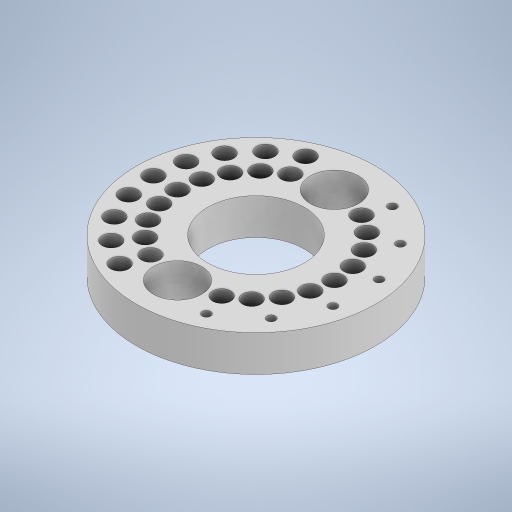
# Autodesk Inventor part: top_housing_wire_guide
Saved by Autodesk Inventor 2023.1 (Build 271208000, 208)
## iProperties
Created: 2026-04-22
Part Number: top_housing_wire_guide
Material: Generic
Document SubType Name: Modeling
Designer: Lars
Density: 1 g/cm^3
Appearance: Default
Author: Lars
Autodesk Inventor part; units mm, degrees
ref_plane "YZ Plane" through (0, 0, 0) normal (1, 0, 0) x (0, 1, 0)
ref_plane "XZ Plane" through (0, 0, 0) normal (0, 1, 0) x (-1, 0, 0)
ref_plane "XY Plane" through (0, 0, 0) normal (0, 0, 1) x (1, 0, 0)
sketch "Sketch2" plane through (0, 0, 0) normal (0, 1, 0) x (-1, 0, 0)
  circle A0 centre (0, 0) radius 10 construction
  circle A1 centre (0, 0) radius 9.9
  circle A2 centre (0, 0) radius 5 construction
  circle A3 centre (0, 0) radius 7 construction
  point P0 (0, 7)
  dimension "d8" = 14
  dimension "d5" = 20
  dimension "d6" = 0.1
  dimension "d7" = 10
  constraints: 3 centre point, 3 coincident, 2 vertical alignment, 2 other
  measures "d5" diameter of A0
  measures "d6" radial gap between concentric circles of A0 A1
  measures "d7" diameter of A2
extrude "Extrusion1" add sketch "Sketch2" along normal blind 3
sketch "Sketch3" plane through (0, 3, 0) normal (0, 1, 0) x (1, 0, 0)
  circle A0 centre (0, 0) radius 6.5 construction
  circle A1 centre (-6.5, 0) radius 0.75
  circle A2 centre (0, 0) radius 4
  circle A3 centre (0, 0) radius 8.5 construction
  circle A4 centre (0, -6.5) radius 2
  circle A5 centre (0, 6.5) radius 2
  circle A6 centre (-6.256, 1.7644) radius 0.75
  circle A7 centre (-5.5422, 3.3962) radius 0.75
  circle A8 centre (-4.4122, 4.7731) radius 0.75
  circle A9 centre (-2.9509, 5.7915) radius 0.75
  circle A10 centre (-6.256, -1.7644) radius 0.75
  circle A11 centre (-5.5422, -3.3962) radius 0.75
  circle A12 centre (-4.4122, -4.7731) radius 0.75
  circle A13 centre (-2.9509, -5.7915) radius 0.75
  circle A14 centre (-8.5, 0) radius 0.75
  circle A15 centre (-8.1604, -2.3785) radius 0.75
  circle A16 centre (-7.1688, -4.567) radius 0.75
  circle A17 centre (-5.6044, -6.3906) radius 0.75
  circle A18 centre (-3.5923, -7.7036) radius 0.75
  circle A19 centre (-8.1604, 2.3785) radius 0.75
  circle A20 centre (-7.1688, 4.567) radius 0.75
  circle A21 centre (-5.6044, 6.3906) radius 0.75
  circle A22 centre (-3.5923, 7.7036) radius 0.75
  circle A23 centre (0, 0) radius 9.9 projected
  line L0 (0, -9.9) -> (0, 9.9) construction
  circle A24 centre (6.5, 0) radius 0.75
  circle A25 centre (6.256, 1.7644) radius 0.75
  circle A26 centre (5.5422, 3.3962) radius 0.75
  circle A27 centre (4.4122, 4.7731) radius 0.75
  circle A28 centre (2.9509, 5.7915) radius 0.75
  circle A29 centre (6.256, -1.7644) radius 0.75
  circle A30 centre (5.5422, -3.3962) radius 0.75
  circle A31 centre (4.4122, -4.7731) radius 0.75
  circle A32 centre (2.9509, -5.7915) radius 0.75
  arc A33 (3.5923, -7.7036) -> (8.5, 0) centre (0, 0) ccw construction
  circle A34 centre (3.5923, -7.7036) radius 0.35
  circle A35 centre (6.6057, -5.3492) radius 0.35
  circle A36 centre (8.2821, -1.9121) radius 0.35
  circle A37 centre (8.2821, 1.9121) radius 0.35
  circle A38 centre (6.6057, 5.3492) radius 0.35
  circle A39 centre (3.5923, 7.7036) radius 0.35
  dimension "d14" = 13
  dimension "d15" = 1.5
  dimension "d16" = 8
  dimension "d17" = 17
  dimension "d18" = 4
  dimension "d19" = 4
  dimension "d22" = 63
  dimension "d26" = 63
  dimension "d28" = 1.5
  dimension "d31" = 65
  dimension "d35" = 65
  dimension "d37" = 0.7
  dimension "d40" = 130
  constraints: 39 centre point, 10 point on circle, 9 symmetric about line, 4 coincident, 2 end point, 1 concentric, 1 vertical, 56 other
  measures "d14" diameter of A0
  measures "d15" diameter of A1
  measures "d16" diameter of A2
  measures "d17" diameter of A3
  measures "d18" diameter of A4
  measures "d19" diameter of A5
  measures "d28" diameter of A14
  measures "d37" diameter of A34
extrude "Extrusion2" cut sketch "Sketch3" against normal blind 3 contours A1 | A2 | A4 | A5 | A6 | A7 | A8 | A9 | A10 | A11 | A12 | A13 | A14 | A15 | A16 | A17 | A18 | A19 | A20 | A21 | A22 | A24 | A25 | A26 | A27 | A28 | A29 | A30 | A31 | A32 | A34 | A35 | A36 | A37 | A38 | A39
body "Solid1"
